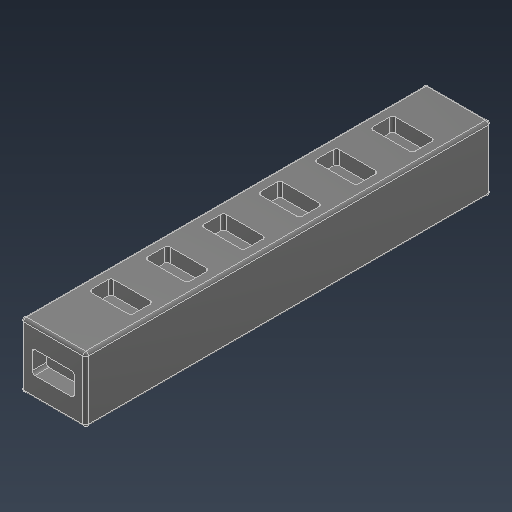
# Autodesk Inventor part: U2H-Z7SBK
Saved by Autodesk Inventor 2021 (Build 250183000, 183)
## iProperties
Created: 2021-07-22
Part Number: U2H-Z7SBK
Material: ABS プラスチック
Document SubType Name: Modeling
Designer: yuta0
Density: 1.06 g/cm^3
Appearance: 滑らか - 黒
購入先: Amazon
在庫数: 0.0
Author: yuta0
Autodesk Inventor part; units mm, degrees
ref_plane "YZ Plane" through (0, 0, 0) normal (1, 0, 0) x (0, 1, 0)
ref_plane "XZ Plane" through (0, 0, 0) normal (0, 1, 0) x (-1, 0, 0)
ref_plane "XY Plane" through (0, 0, 0) normal (0, 0, 1) x (1, 0, 0)
sketch "スケッチ1" plane through (0, 0, 0) normal (0, 0, 1) x (1, 0, 0)
  line L0 (-11.5, -11.5) -> (11.5, -11.5)
  line L1 (11.5, -11.5) -> (11.5, 11.5)
  line L2 (11.5, 11.5) -> (-11.5, 11.5)
  line L3 (-11.5, 11.5) -> (-11.5, -11.5)
  line L4 (-11.5, -11.5) -> (11.5, 11.5) construction
  line L5 (11.5, -11.5) -> (-11.5, 11.5) construction
  point P0 (0, 0)
  dimension "d0" = 23
  dimension "d1" = 23
  constraints: 12 end point, 2 midpoint, 2 parallel, 1 horizontal, 1 perpendicular
  measures "d0" distance of L2.end L1.end
  measures "d1" distance of L1.end L0.end
extrude "押し出し1" add sketch "スケッチ1" along normal mid plane 144
fillet "フィレット1" radius 1 1 edges at (11.5, 0, 72)
fillet "フィレット1" radius 1 12 edges at (-11.5, -11.5, 0) (0, -11.5, 72) (11.5, -11.5, 0) (0, -11.5, -72) (-11.5, 11.5, 0) (-11.5, 0, 72) (-11.5, 0, -72) (11.5, 0, 72) (11.5, 11.5, 0) (11.5, 0, -72) (0, 11.5, 72) (0, 11.5, -72)
sketch "スケッチ2" plane through (0, 0, 72) normal (0, 0, 1) x (1, 0, 0)
  line L0 (-7.5, -4) -> (7.5, -4)
  line L1 (7.5, -4) -> (7.5, 4)
  line L2 (7.5, 4) -> (-7.5, 4)
  line L3 (-7.5, 4) -> (-7.5, -4)
  line L4 (-7.5, -4) -> (7.5, 4) construction
  line L5 (7.5, -4) -> (-7.5, 4) construction
  point P0 (0, 0)
  dimension "d6" = 15
  dimension "d7" = 8
  constraints: 12 end point, 2 midpoint, 2 parallel, 1 horizontal, 1 perpendicular
  measures "d6" distance of L2.end L1.end
  measures "d7" distance of L1.end L0.end
extrude "押し出し2" cut sketch "スケッチ2" against normal blind 5
sketch "スケッチ3" plane through (-10.5, 11.5, -71) normal (0, 1, 0) x (1, 0, 0)
  line L0 (18, -115) -> (3, -115)
  line L1 (3, -115) -> (3, -123)
  line L2 (3, -123) -> (18, -123)
  line L3 (18, -123) -> (18, -115)
  line L4 (18, -115) -> (3, -123) construction
  line L5 (3, -115) -> (18, -123) construction
  line L6 (18, -95) -> (3, -95)
  line L7 (3, -95) -> (3, -103)
  line L8 (3, -103) -> (18, -103)
  line L9 (18, -103) -> (18, -95)
  line L10 (18, -95) -> (3, -103) construction
  line L11 (3, -95) -> (18, -103) construction
  line L12 (18, -75) -> (3, -75)
  line L13 (3, -75) -> (3, -83)
  line L14 (3, -83) -> (18, -83)
  line L15 (18, -83) -> (18, -75)
  line L16 (18, -75) -> (3, -83) construction
  line L17 (3, -75) -> (18, -83) construction
  line L18 (18, -55) -> (3, -55)
  line L19 (3, -55) -> (3, -63)
  line L20 (3, -63) -> (18, -63)
  line L21 (18, -63) -> (18, -55)
  line L22 (18, -55) -> (3, -63) construction
  line L23 (3, -55) -> (18, -63) construction
  line L24 (18, -35) -> (3, -35)
  line L25 (3, -35) -> (3, -43)
  line L26 (3, -43) -> (18, -43)
  line L27 (18, -43) -> (18, -35)
  line L28 (18, -35) -> (3, -43) construction
  line L29 (3, -35) -> (18, -43) construction
  line L30 (18, -15) -> (3, -15)
  line L31 (3, -15) -> (3, -23)
  line L32 (3, -23) -> (18, -23)
  line L33 (18, -23) -> (18, -15)
  line L34 (18, -15) -> (3, -23) construction
  line L35 (3, -15) -> (18, -23) construction
  line L36 (21, 1) -> (0, 1) projected
  line L37 (-1, 0) -> (-1, -142) projected
  point P0 (10.5, -71)
  point P1 (10.5, -119)
  point P2 (10.5, -99)
  point P3 (10.5, -79)
  point P4 (10.5, -59)
  point P5 (10.5, -39)
  point P6 (10.5, -19)
  dimension "d10" = 15
  dimension "d11" = 8
  dimension "d14" = 20
  dimension "d19" = 20
  dimension "d20" = 11.5
  constraints: 72 end point, 12 midpoint, 2 parallel, 1 collinear, 1 horizontal, 1 perpendicular, 1 vertical, 54 other
  measures "d10" distance of L2.end L1.end
  measures "d11" distance of L1.end L0.end
  measures "d14" distance of L0.start L6.start
  measures "d19" distance from line of L36 point (10.5, -19)
  measures "d20" distance from line of point (10.5, -119) L37
extrude "押し出し3" cut sketch "スケッチ3" against normal blind 5
sketch "スケッチ4" plane through (0, 0, -72) normal (0, 0, -1) x (-1, 0, 0)
  line L0 (0.5, -5) -> (5.5, -5)
  line L1 (5.5, -5) -> (5.5, -1)
  line L2 (5.5, -1) -> (0.5, -1)
  line L3 (0.5, -1) -> (0.5, -5)
  line L4 (0.5, -5) -> (5.5, -1) construction
  line L5 (5.5, -5) -> (0.5, -1) construction
  point P0 (0, 0)
  point P1 (3, -3)
  dimension "d23" = 5
  dimension "d24" = 4
  dimension "d25" = 3
  dimension "d26" = 3
  constraints: 12 end point, 2 midpoint, 2 parallel, 1 horizontal, 1 perpendicular
  measures "d23" distance of L1.end L2.end
  measures "d24" distance of L2.end L0.start
  measures "d25" horizontal distance of point (0, 0) point (3, -3)
  measures "d26" horizontal distance of point (0, 0) point (3, -3)
extrude "押し出し4" cut sketch "スケッチ4" against normal blind 3
fillet "フィレット2" radius 1 28 edges at (-7.5, 9, -56) (7.5, 9, -56) (7.5, 9, -48) (-7.5, 9, -48) (-7.5, 9, -36) (7.5, 9, -36) (7.5, 9, -28) (-7.5, 9, -28) (-7.5, 9, -16) (-7.5, 9, -8) (7.5, 9, -8) (7.5, 9, -16) (-7.5, 9, 4) (7.5, 9, 4) (7.5, 9, 12) (-7.5, 9, 12) (-7.5, 9, 24) (-7.5, 9, 32) (7.5, 9, 32) (7.5, 9, 24) (-7.5, 9, 44) (-7.5, 9, 52) (7.5, 9, 52) (7.5, 9, 44) (-7.5, -4, 69.5) (-7.5, 4, 69.5) (7.5, 4, 69.5) (7.5, -4, 69.5)
